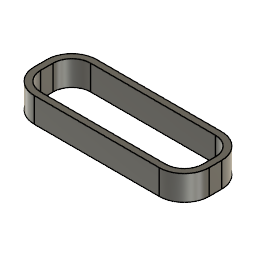
controller (Autodesk Fusion 360 archive; units mm, degrees)
design "base"
part number: 2026-06-19-17-07-45-860
Autodesk Fusion 360 part; units mm, degrees
sketch "Szkic1" plane through (0, 0, 0) normal (0, 0, 1) x (1, 0, 0)
  line L0 (20, 0) -> (120, 0)
  line L1 (140, 20) -> (140, 30)
  line L2 (0, 20) -> (0, 30)
  line L3 (20, 50) -> (120, 50)
  arc A0 (0, 20) -> (20, 0) centre (20, 20) ccw
  arc A1 (20, 50) -> (0, 30) centre (20, 30) ccw
  arc A2 (140, 30) -> (120, 50) centre (120, 30) ccw
  arc A3 (120, 0) -> (140, 20) centre (120, 20) ccw
  line L4 (20, 5) -> (120, 5)
  line L5 (135, 20) -> (135, 30)
  line L6 (120, 45) -> (20, 45)
  line L7 (5, 30) -> (5, 20)
  arc A4 (20, 45) -> (5, 30) centre (20, 30) ccw
  arc A5 (5, 20) -> (20, 5) centre (20, 20) ccw
  arc A6 (135, 30) -> (120, 45) centre (120, 30) ccw
  arc A7 (120, 5) -> (135, 20) centre (120, 20) ccw
  point P0 (140, 0)
  point P1 (140, 50)
  point P2 (135, 5)
  point P3 (135, 45)
  point P4 (5, 45)
  constraint horizontal L0
  constraint perpendicular L0 L1
  constraint perpendicular L0 L2
  constraint perpendicular L1 L3
  constraint coincident origin L0
  constraint tangent L0 A0
  constraint tangent L2 A0
  constraint tangent L2 A1
  constraint tangent L3 A1
  constraint coincident P1 L3
  constraint coincident P1 L1
  constraint tangent L3 A2
  constraint tangent L1 A2
  constraint coincident P0 L0
  constraint coincident P0 L1
  constraint tangent L0 A3
  constraint tangent L1 A3
  constraint parallel L0 L4
  constraint perpendicular L4 L5
  constraint perpendicular L5 L6
  constraint perpendicular L4 L7
  constraint coincident P4 L7
  constraint coincident P4 L6
  constraint tangent L7 A4
  constraint tangent L6 A4
  constraint tangent L7 A5
  constraint tangent L4 A5
  constraint coincident P3 L6
  constraint coincident P3 L5
  constraint tangent L6 A6
  constraint tangent L5 A6
  constraint coincident P2 L4
  constraint coincident P2 L5
  constraint tangent L4 A7
  constraint tangent L5 A7
extrude "Wyciągnięcie proste1" add sketch "Szkic1" along normal blind 20

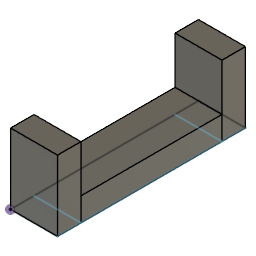
design "bridge"
part number: 2026-06-19-19-02-43-658
Autodesk Fusion 360 part; units mm, degrees
sketch "Szkic1" plane through (0, 0, 0) normal (0, 0, 1) x (1, 0, 0)
  line L0 (0, 0) -> (10, 0)
  line L1 (10, 0) -> (10, 40)
  line L2 (0, 0) -> (0, 40)
  line L3 (0, 40) -> (10, 40)
  line L4 (0, 5) -> (10, 5)
  line L5 (0, 35) -> (10, 35)
  dimension "d3" = 40
  constraint coincident L0.start L2.start
  constraint horizontal L0
  constraint perpendicular L0 L1
  constraint perpendicular L0 L2
  constraint perpendicular L1 L3
  constraint coincident L2 L4.start
  constraint coincident L1 L4.end
  constraint perpendicular L1 L4
  constraint coincident L2 L5.start
  constraint coincident L1 L5.end
  constraint perpendicular L1 L5
  measures "d3" distance of L0.start L2.end
extrude "Wyciągnięcie proste1" add sketch "Szkic1" along normal blind 15 contours L0 L1 L2 L4 | L1 L2 L3 L5 makes body 1 at (3.3333, 40, 5) makes body 2 at (3.3333, 5, 5)
extrude "Wyciągnięcie proste2" add sketch "Szkic1" along normal blind 5 separate body contours L1 L2 L4 L5 makes body 3
